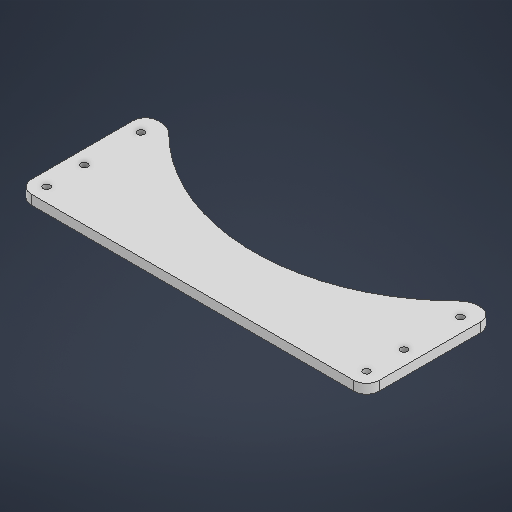
# Autodesk Inventor part: Intake (Plastic)
Saved by Autodesk Inventor 2025 (Build 290162000, 162)
## iProperties
Created: 2024-12-30
Part Number: Intake (Plastic)
Material: Generic
Document SubType Name: Modeling
Designer: Juan
Density: 1 g/cm^3
Appearance: Default
Author: Juan
Autodesk Inventor part; units mm, degrees
ref_plane "YZ Plane" through (0, 0, 0) normal (1, 0, 0) x (0, 1, 0)
ref_plane "XZ Plane" through (0, 0, 0) normal (0, 1, 0) x (-1, 0, 0)
ref_plane "XY Plane" through (0, 0, 0) normal (0, 0, 1) x (1, 0, 0)
sketch "Sketch1" plane through (0, 0, 0) normal (0, 1, 0) x (-1, 0, 0)
  line L0 (0, 0) -> (-228.6, 0)
  line L1 (-228.6, 0) -> (-228.6, -82.55)
  line L2 (0, 0) -> (0, -82.55)
  line L3 (-228.6, 0) -> (-222.25, 0)
  circle A0 centre (-222.25, -6.35) radius 2.3241
  circle A1 centre (-222.25, -31.75) radius 2.3241
  line L4 (-228.6, 0) -> (-114.3, 0)
  line L5 (-114.3, 0) -> (-114.3, 9.4502)
  circle A2 centre (-222.25, -69.85) radius 2.3241
  circle A3 centre (-6.35, -6.35) radius 2.3241
  circle A4 centre (-6.35, -31.75) radius 2.3241
  circle A5 centre (-6.35, -69.85) radius 2.3241
  line L6 (-228.6, -82.55) -> (-215.9, -82.55)
  line L7 (0, -82.55) -> (-12.7, -82.55)
  line L8 (-114.3, 0) -> (-114.3, -38.1)
  arc A6 (-12.7, -82.55) -> (-215.9, -82.55) centre (-114.3, -176.4393) ccw
  line L9 (-228.6, 0) -> (-231.775, 0)
  line L10 (-231.775, 0) -> (-231.775, -82.55)
  line L11 (-231.775, -82.55) -> (-228.6, -82.55)
  line L12 (-228.6, 0) -> (-228.6, 3.175)
  line L13 (-228.6, 3.175) -> (-231.775, 3.175)
  line L14 (-231.775, 3.175) -> (-231.775, 0)
  line L15 (-228.6, 3.175) -> (0, 3.175)
  line L16 (0, 3.175) -> (0, 0)
  line L17 (0, 0) -> (3.175, 0)
  line L18 (3.175, 0) -> (3.175, 3.175)
  line L19 (3.175, 3.175) -> (0, 3.175)
  line L20 (3.175, 0) -> (3.175, -82.55)
  line L21 (3.175, -82.55) -> (0, -82.55)
  point P0 (-225.425, 0)
  dimension "d0" = 228.6
  dimension "d1" = 82.55
  dimension "d2" = 6.35
  dimension "d4" = 4.6482
  dimension "d6" = 4.6482
  dimension "d7" = 114.3
  dimension "d9" = 4.6482
  dimension "d10" = 6.35
  dimension "d11" = 31.75
  dimension "d12" = 69.85
  dimension "d14" = 12.7
  dimension "d15" = 12.7
  dimension "d16" = 38.1
  dimension "d20" = 3.175
  dimension "d21" = 3.175
  dimension "d22" = 3.175
  constraints: 44 end point, 8 perpendicular, 7 centre point, 4 point on line, 4 vertical, 3 horizontal, 3 point on circle, 3 symmetric about line, 2 collinear, 2 midpoint, 1 parallel, 3 other
  measures "d0" distance of L0.start L0.end
  measures "d1" distance of L0.end L1.end
  measures "d2" distance of L0.end L3.end
  measures "d4" diameter of A0
  measures "d6" diameter of A1
  measures "d7" distance of L0.end L4.end
  measures "d9" diameter of A2
  measures "d10" distance from line of A0.centre L0
  measures "d11" distance from line of L0 A1.centre
  measures "d12" vertical distance of point (-225.425, 0) A2.centre
  measures "d14" distance of L1.end L6.end
  measures "d15" distance of L2.end L7.end
  measures "d16" distance of L4.end L8.end
  measures "d20" distance of L0.end L9.end
  measures "d21" distance of L0.end L12.end
  measures "d22" distance of L0.start L17.end
extrude "Extrusion1" add sketch "Sketch1" against normal blind 3.175 contours L2 L7 A6 L8 L0 | L8 A6 L6 L1 L0
fillet "Fillet1" radius 8.4667 4 edges at (228.6, -1.5875, -82.55) (215.9, -1.5875, -82.55) (12.7, -1.5875, -82.55) (0, -1.5875, -82.55)
extrude "Extrusion2" add sketch "Sketch1" against normal blind 6.35
fillet "Fillet2" radius 8.4667 4 edges at (231.775, -3.175, -82.55) (231.775, -3.175, 3.175) (-3.175, -3.175, 3.175) (-3.175, -3.175, -82.55)
fillet "Fillet3" radius 12.7 2 edges at (215.9, -3.175, -82.55) (12.7, -3.175, -82.55)
body "Solid1"
